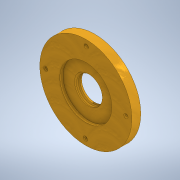
# Autodesk Inventor part: Круг основание
Saved by Autodesk Inventor 2020 (Build 240168000, 168)
## iProperties
Created: 2021-04-21
Part Number: Круг основание
Material: Латунь, мягкая, желтая, сварочная
Document SubType Name: Modeling
Designer: lbfas
Density: 8.5 g/cm^3
Appearance: Сварка — латунь
Author: lbfas
Autodesk Inventor part; units mm, degrees
ref_plane "YZ Plane" through (0, 0, 0) normal (1, 0, 0) x (0, 1, 0)
sketch "Эскиз1" plane through (0, 0, 0) normal (0, 0, 1) x (1, 0, 0)
  circle A0 centre (0, 0) radius 43.75
  dimension "d0" = 87.5
  constraints: 1 centre point, 1 coincident
  measures "d0" diameter of A0
extrude "Выдавливание1" add sketch "Эскиз1" along normal blind 8.5
sketch "Эскиз2" plane through (0, 0, 8.5) normal (0, 0, 1) x (1, 0, 0)
  circle A0 centre (0, 0) radius 24.75
  dimension "d3" = 49.5
  constraints: 1 centre point, 1 coincident
  measures "d3" diameter of A0
extrude "Выдавливание2" cut sketch "Эскиз2" against normal blind 3
sketch "Эскиз3" plane through (0, 0, 5.5) normal (0, 0, 1) x (1, 0, 0)
  circle A0 centre (0, 0) radius 12.5
  dimension "d6" = 25
  constraints: 1 centre point, 1 coincident
  measures "d6" diameter of A0
extrude "Выдавливание3" cut sketch "Эскиз3" against normal blind 50
sketch "Эскиз7" plane through (0, 0, 0) normal (0, 0, -1) x (-1, 0, 0)
  line L0 (0, 0) -> (-38, 0)
  circle A0 centre (-38, 0) radius 1.5
  dimension "d82" = 38
  dimension "d83" = 3
  constraints: 2 end point, 1 centre point, 1 coincident, 1 horizontal
  measures "d82" distance of L0.start L0.end
  measures "d83" diameter of A0
extrude "Выдавливание5" cut sketch "Эскиз7" against normal blind 10
pattern_circular "Круговой массив4" count 4 over 360 about axis through (0, 0, 5.5) along (0, 0, -1) of "Выдавливание5"
ref_plane "РабПлоскость4" through (38, 0, 0) normal (0.7265681, -0.6870944, 0) x (0.6870944, 0.7265681, 0)
sketch "Эскиз9" plane through (38, 0, 0) normal (0.7265681, -0.6870944, 0) x (0.6870944, 0.7265681, 0)
  line L0 (1.5, 0) -> (1.5, 8.5) projected
  line L1 (1.5, 3.0774) -> (2.5, 3.0774)
  line L2 (17.6404, 8.5) -> (-69.8596, 8.5) projected
  line L3 (2.5, 3.0774) -> (1.5, 3.6547)
  line L4 (1.5, 3.0774) -> (1.5, 3.6547)
  line L5 (2.5, 3.0774) -> (1.5, 2.5)
  line L6 (1.5, 3.0774) -> (1.5, 2.5)
  line L7 (1.5, 0) -> (1.5, 2.5)
  point P0 (-26.1096, 0)
  dimension "d102" = 1
  dimension "d103" = 30
  dimension "d104" = 2.5
  constraints: 12 end point, 1 point on line, 1 symmetric about line, 1 other
  measures "d102" distance of L1.start L1.end
  measures "d103" angle of L3 L1
  measures "d104" distance of L0.start L7.end
coil "Пружина7" sketch "Эскиз9" operation cut axis through (38, 0, 0) along (0, 0, 1) pitch 1.155 turns 8.658009 hand right
chamfer "Фаска6" distance 2.5 angle 45 1 edges at (39.5, 0, 0)
pattern_circular "Круговой массив5" count 4 over 360 about axis through (0, 0, 5.5) along (0, 0, -1) of "Пружина7"
chamfer "Фаска9" distance 2.5 angle 45 3 edges at (0, -39.5, 0) (-39.5, 0, 0) (0, 39.5, 0)
ref_plane "РабПлоскость5" through (0, 0, 5.5) normal (0.9992206, -0.0394737, 0) x (0.0394737, 0.9992206, 0)
sketch "Эскиз10" plane through (0, 0, 5.5) normal (0.9992206, -0.0394737, 0) x (0.0394737, 0.9992206, 0)
  line L0 (12.5, -5.5) -> (-12.5, -5.5) projected
  line L1 (-12.5, -4.634) -> (-14, -4.634)
  line L2 (43.75, -5.5) -> (-43.75, -5.5) projected
  line L3 (-14, -4.634) -> (-12.5, -5.5)
  line L4 (-12.5, -4.634) -> (-12.5, -5.5)
  line L5 (-14, -4.634) -> (-12.5, -3.768)
  line L6 (-12.5, -4.634) -> (-12.5, -3.768)
  point P0 (0, -5.5)
  dimension "d128" = 1.732
  dimension "d129" = 30
  constraints: 10 end point, 1 symmetric about line, 1 vertical
  measures "d128" distance of L0.end L1.end
  measures "d129" angle of L3 L1
coil "Пружина8" sketch "Эскиз10" operation cut axis through (0, 0, 5.5) along (0, 0, 1) pitch 1.732 turns 5.773672 hand right
